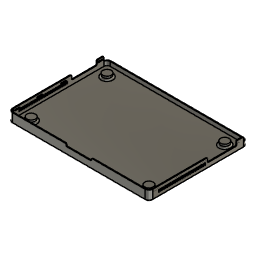
macbook case v2 (Autodesk Fusion 360 design; units mm, degrees)
Autodesk Fusion 360 part; units mm, degrees
note: some values were not read from the file. Chosen so that the rebuilt part matches the saved one: which bodies a step acts on.
sketch "Sketch1" plane through (0, 0, 0) normal (0, 0, 1) x (1, 0, 0)
  line L0 (93.5786, -68.8674) -> (-266.4214, -68.8674)
  line L1 (-266.4214, -68.8674) -> (-266.4214, 183.6326)
  line L2 (-266.4214, 183.6326) -> (93.5786, 183.6326)
  line L3 (93.5786, 183.6326) -> (93.5786, -68.8674)
  dimension "d1" = 360
  dimension "d2" = 252.5
  constraint horizontal L0
  constraint vertical L1
  constraint horizontal L2
  constraint vertical L3
  measures "d1" distance of L0.start L0.end
  measures "d2" distance of L0.start L2.end
extrude "Extrude1" add sketch "Sketch1" along normal blind 12.4 makes body 1
fillet "Fillet1" radius 10 4 edges at (-266.4214, 183.6326, 6.2) (-266.4214, -68.8674, 6.2) (93.5786, -68.8674, 6.2) (93.5786, 183.6326, 6.2) on bodies 1
shell "Shell1" thickness 2 removed faces 1 at (-143.0881, 99.466, 12.4) on bodies 1
chamfer "Chamfer1" distance 2 angle 45 8 edges at (93.5786, 57.3826, 0) (90.6497, -65.9384, 0) (-86.4214, -68.8674, 0) (-263.4925, -65.9384, 0) (-266.4214, 57.3826, 0) (-263.4925, 180.7037, 0) (-86.4214, 183.6326, 0) (90.6497, 180.7037, 0) on bodies 1
extrude "Extrude2" add 1 faces at (-29.7547, -68.2007, 12.4) along direction (0, 0, 1) blind 13 on bodies 1 bodies 1
sketch "Sketch2" plane through (0, 183.6326, 0) normal (0, 1, 0) x (-1, 0, 0)
  line L0 (-83.5786, 2) -> (256.4214, 2)
  line L1 (256.4214, 2) -> (256.4214, 25.4)
  line L2 (256.4214, 25.4) -> (-83.5786, 25.4)
  line L3 (-83.5786, 25.4) -> (-83.5786, 2)
  line L4 (-113.9565, 25.4) -> (284.3902, 25.4)
  line L5 (284.3902, 25.4) -> (284.3902, 13)
  line L6 (284.3902, 13) -> (-113.9565, 13)
  line L7 (-113.9565, 13) -> (-113.9565, 25.4)
  dimension "d11" = 12.4
  constraint horizontal L4
  constraint vertical L5
  constraint horizontal L6
  constraint vertical L7
  measures "d11" distance of L4.start L6.end
extrude "Extrude3" cut sketch "Sketch2" against normal blind 10 contours L3 L4 L6 L7 | L1 L2 L3 L4 L6 | L1 L4 L5 L6 bodies 1
sketch "Sketch3" plane through (-266.4214, 0, 0) normal (-1, 0, 0) x (0, -1, 0)
  line L0 (-173.6326, 2) -> (58.8674, 2)
  line L1 (58.8674, 2) -> (58.8674, 25.4)
  line L2 (58.8674, 25.4) -> (-173.6326, 25.4)
  line L3 (-173.6326, 25.4) -> (-173.6326, 13)
  line L4 (-173.6326, 13) -> (-173.6326, 2)
  line L5 (68.8674, 2) -> (68.8674, 25.4)
  line L6 (68.8674, 25.4) -> (-156.1326, 25.4) construction
  line L7 (-156.1326, 25.4) -> (-86.1326, 25.4)
  line L8 (-86.1326, 25.4) -> (-86.1326, 13)
  line L9 (-86.1326, 13) -> (-156.1326, 13)
  line L10 (-156.1326, 13) -> (-156.1326, 25.4)
  dimension "d14" = 225
  dimension "d15" = 70
  dimension "d16" = 12.4
  constraint coincident L5.end L6.start
  constraint perpendicular L1 L6
  constraint horizontal L7
  constraint vertical L8
  constraint horizontal L9
  constraint vertical L10
  measures "d14" distance of L5.end L6.end
  measures "d15" distance of L6.end L7.end
  measures "d16" distance of L6.end L9.end
extrude "Extrude4" cut sketch "Sketch3" against normal blind 30 contours L2 L7 L8 L9 L10 bodies 1
sketch "Sketch4" plane through (93.5786, 0, 0) normal (1, 0, 0) x (0, 1, 0)
  line L0 (-58.8674, 2) -> (173.6326, 2)
  line L1 (173.6326, 2) -> (173.6326, 13)
  line L2 (173.6326, 13) -> (173.6326, 25.4)
  line L3 (173.6326, 25.4) -> (-58.8674, 25.4)
  line L4 (-58.8674, 25.4) -> (-58.8674, 2)
  line L5 (-68.8674, 25.4) -> (-68.8674, 2)
  line L6 (-68.8674, 25.4) -> (156.1326, 25.4) construction
  line L7 (156.1326, 25.4) -> (81.1326, 25.4)
  line L8 (81.1326, 25.4) -> (81.1326, 13)
  line L9 (81.1326, 13) -> (156.1326, 13)
  line L10 (156.1326, 13) -> (156.1326, 25.4)
  dimension "d19" = 225
  dimension "d20" = 75
  dimension "d21" = 12.4
  constraint coincident L5.start L6.start
  constraint perpendicular L5 L6
  constraint horizontal L7
  constraint vertical L8
  constraint horizontal L9
  constraint vertical L10
  measures "d19" distance of L5.start L6.end
  measures "d20" distance of L6.end L7.end
  measures "d21" distance of L6.end L9.end
extrude "Extrude5" cut sketch "Sketch4" against normal blind 30 contours L3 L7 L8 L9 L10 bodies 1
sketch "Sketch5" plane through (93.5786, 0, 0) normal (1, 0, 0) x (0, 1, 0)
  line L0 (156.1326, 25.4) -> (156.1326, 13)
  line L1 (156.1326, 13) -> (81.1326, 13)
  line L2 (81.1326, 13) -> (81.1326, 25.4)
  line L3 (81.1326, 25.4) -> (-58.8674, 25.4)
  line L4 (-58.8674, 25.4) -> (-58.8674, 2)
  line L5 (-58.8674, 2) -> (173.6326, 2)
  line L6 (173.6326, 2) -> (173.6326, 13)
  line L7 (173.6326, 13) -> (173.6326, 25.4)
  line L8 (173.6326, 25.4) -> (156.1326, 25.4)
  line L9 (-68.8674, 25.4) -> (-68.8674, 2)
  line L10 (-68.8674, 25.4) -> (81.1326, 25.4) construction
  line L11 (6.1326, 25.4) -> (6.1326, 15.9) construction
  line L12 (-43.8674, 15.9) -> (81.1326, 15.9)
  line L13 (81.1326, 15.9) -> (81.1326, 9.9)
  line L14 (81.1326, 9.9) -> (-43.8674, 9.9)
  line L15 (-43.8674, 9.9) -> (-43.8674, 15.9)
  line L16 (-68.8674, 15.9) -> (-43.8674, 15.9) construction
  line L17 (-43.8674, 15.9) -> (-41.8674, 15.9)
  line L18 (-41.8674, 15.9) -> (-41.8674, 9.9)
  line L19 (-41.8674, 9.9) -> (-43.8674, 9.9)
  line L20 (-43.8674, 9.9) -> (-43.8674, 15.9)
  dimension "d24" = 150
  dimension "d25" = 9.5
  dimension "d26" = 125
  dimension "d27" = 6
  dimension "d28" = 25
  dimension "d29" = 2
  constraint coincident L9.start L10.start
  constraint perpendicular L4 L10
  constraint midpoint L10 L11.start
  constraint perpendicular L5 L11
  constraint horizontal L12
  constraint vertical L13
  constraint horizontal L14
  constraint vertical L15
  constraint coincident L9 L16.start
  constraint perpendicular L4 L16
  constraint coincident L12.start L15.end
  constraint horizontal L17
  constraint vertical L18
  constraint horizontal L19
  constraint vertical L20
  measures "d24" distance of L9.start L2.end
  measures "d25" distance of L11.start L11.end
  measures "d26" distance of L12.start L12.end
  measures "d27" distance of L12.start L14.end
  measures "d28" distance of L16.start L12.start
  measures "d29" distance of L12.start L17.end
extrude "Extrude6" cut sketch "Sketch5" against normal blind 460 contours L12 L14 L15 L17 L18 L19 L20 bodies 1
pattern_linear "R-Pattern1" count 30 spacing 4.2069 along (0, 1, 0) of "Extrude6"
extrude "Extrude7" add 1 faces at (-265.7547, 86.1326, 21.2667) along direction (0, 1, 0) blind 5 on bodies 1 bodies 1
sketch "Sketch6" plane through (93.5786, 0, 0) normal (1, 0, 0) x (0, 1, 0)
  line L0 (80.1326, 15.9) -> (80.1326, 9.9)
  line L1 (80.1326, 9.9) -> (78.1326, 9.9)
  line L2 (78.1326, 9.9) -> (78.1326, 15.9)
  line L3 (78.1326, 15.9) -> (80.1326, 15.9)
  line L4 (75.9257, 15.9) -> (75.9257, 9.9)
  line L5 (75.9257, 9.9) -> (73.9257, 9.9)
  line L6 (73.9257, 9.9) -> (73.9257, 15.9)
  line L7 (73.9257, 15.9) -> (75.9257, 15.9)
  line L8 (71.7188, 15.9) -> (71.7188, 9.9)
  line L9 (71.7188, 9.9) -> (69.7188, 9.9)
  line L10 (69.7188, 9.9) -> (69.7188, 15.9)
  line L11 (69.7188, 15.9) -> (71.7188, 15.9)
  line L12 (67.5119, 15.9) -> (67.5119, 9.9)
  line L13 (67.5119, 9.9) -> (65.5119, 9.9)
  line L14 (65.5119, 9.9) -> (65.5119, 15.9)
  line L15 (65.5119, 15.9) -> (67.5119, 15.9)
  line L16 (63.305, 15.9) -> (63.305, 9.9)
  line L17 (63.305, 9.9) -> (61.305, 9.9)
  line L18 (61.305, 9.9) -> (61.305, 15.9)
  line L19 (61.305, 15.9) -> (63.305, 15.9)
  line L20 (59.0981, 15.9) -> (59.0981, 9.9)
  line L21 (59.0981, 9.9) -> (57.0981, 9.9)
  line L22 (57.0981, 9.9) -> (57.0981, 15.9)
  line L23 (57.0981, 15.9) -> (59.0981, 15.9)
  line L24 (54.8912, 15.9) -> (54.8912, 9.9)
  line L25 (54.8912, 9.9) -> (52.8912, 9.9)
  line L26 (52.8912, 9.9) -> (52.8912, 15.9)
  line L27 (52.8912, 15.9) -> (54.8912, 15.9)
  line L28 (50.6844, 15.9) -> (50.6844, 9.9)
  line L29 (50.6844, 9.9) -> (48.6844, 9.9)
  line L30 (48.6844, 9.9) -> (48.6844, 15.9)
  line L31 (48.6844, 15.9) -> (50.6844, 15.9)
  line L32 (46.4775, 15.9) -> (46.4775, 9.9)
  line L33 (46.4775, 9.9) -> (44.4775, 9.9)
  line L34 (44.4775, 9.9) -> (44.4775, 15.9)
  line L35 (44.4775, 15.9) -> (46.4775, 15.9)
  line L36 (42.2706, 15.9) -> (42.2706, 9.9)
  line L37 (42.2706, 9.9) -> (40.2706, 9.9)
  line L38 (40.2706, 9.9) -> (40.2706, 15.9)
  line L39 (40.2706, 15.9) -> (42.2706, 15.9)
  line L40 (38.0637, 15.9) -> (38.0637, 9.9)
  line L41 (38.0637, 9.9) -> (36.0637, 9.9)
  line L42 (36.0637, 9.9) -> (36.0637, 15.9)
  line L43 (36.0637, 15.9) -> (38.0637, 15.9)
  line L44 (33.8568, 15.9) -> (33.8568, 9.9)
  line L45 (33.8568, 9.9) -> (31.8568, 9.9)
  line L46 (31.8568, 9.9) -> (31.8568, 15.9)
  line L47 (31.8568, 15.9) -> (33.8568, 15.9)
  line L48 (29.6499, 15.9) -> (29.6499, 9.9)
  line L49 (29.6499, 9.9) -> (27.6499, 9.9)
  line L50 (27.6499, 9.9) -> (27.6499, 15.9)
  line L51 (27.6499, 15.9) -> (29.6499, 15.9)
  line L52 (25.443, 15.9) -> (25.443, 9.9)
  line L53 (25.443, 9.9) -> (23.443, 9.9)
  line L54 (23.443, 9.9) -> (23.443, 15.9)
  line L55 (23.443, 15.9) -> (25.443, 15.9)
  line L56 (21.2361, 15.9) -> (21.2361, 9.9)
  line L57 (21.2361, 9.9) -> (19.2361, 9.9)
  line L58 (19.2361, 9.9) -> (19.2361, 15.9)
  line L59 (19.2361, 15.9) -> (21.2361, 15.9)
  line L60 (17.0292, 15.9) -> (17.0292, 9.9)
  line L61 (17.0292, 9.9) -> (15.0292, 9.9)
  line L62 (15.0292, 9.9) -> (15.0292, 15.9)
  line L63 (15.0292, 15.9) -> (17.0292, 15.9)
  line L64 (12.8223, 15.9) -> (12.8223, 9.9)
  line L65 (12.8223, 9.9) -> (10.8223, 9.9)
  line L66 (10.8223, 9.9) -> (10.8223, 15.9)
  line L67 (10.8223, 15.9) -> (12.8223, 15.9)
  line L68 (8.6154, 15.9) -> (8.6154, 9.9)
  line L69 (8.6154, 9.9) -> (6.6154, 9.9)
  line L70 (6.6154, 9.9) -> (6.6154, 15.9)
  line L71 (6.6154, 15.9) -> (8.6154, 15.9)
  line L72 (4.4085, 15.9) -> (4.4085, 9.9)
  line L73 (4.4085, 9.9) -> (2.4085, 9.9)
  line L74 (2.4085, 9.9) -> (2.4085, 15.9)
  line L75 (2.4085, 15.9) -> (4.4085, 15.9)
  line L76 (0.2016, 15.9) -> (0.2016, 9.9)
  line L77 (0.2016, 9.9) -> (-1.7984, 9.9)
  line L78 (-1.7984, 9.9) -> (-1.7984, 15.9)
  line L79 (-1.7984, 15.9) -> (0.2016, 15.9)
  line L80 (-4.0053, 15.9) -> (-4.0053, 9.9)
  line L81 (-4.0053, 9.9) -> (-6.0053, 9.9)
  line L82 (-6.0053, 9.9) -> (-6.0053, 15.9)
  line L83 (-6.0053, 15.9) -> (-4.0053, 15.9)
  line L84 (-8.2122, 15.9) -> (-8.2122, 9.9)
  line L85 (-8.2122, 9.9) -> (-10.2122, 9.9)
  line L86 (-10.2122, 9.9) -> (-10.2122, 15.9)
  line L87 (-10.2122, 15.9) -> (-8.2122, 15.9)
  line L88 (-12.4191, 15.9) -> (-12.4191, 9.9)
  line L89 (-12.4191, 9.9) -> (-14.4191, 9.9)
  line L90 (-14.4191, 9.9) -> (-14.4191, 15.9)
  line L91 (-14.4191, 15.9) -> (-12.4191, 15.9)
  line L92 (-16.626, 15.9) -> (-16.626, 9.9)
  line L93 (-16.626, 9.9) -> (-18.626, 9.9)
  line L94 (-18.626, 9.9) -> (-18.626, 15.9)
  line L95 (-18.626, 15.9) -> (-16.626, 15.9)
  line L96 (-20.8329, 15.9) -> (-20.8329, 9.9)
  line L97 (-20.8329, 9.9) -> (-22.8329, 9.9)
  line L98 (-22.8329, 9.9) -> (-22.8329, 15.9)
  line L99 (-22.8329, 15.9) -> (-20.8329, 15.9)
  line L100 (-25.0398, 15.9) -> (-25.0398, 9.9)
  line L101 (-25.0398, 9.9) -> (-27.0398, 9.9)
  line L102 (-27.0398, 9.9) -> (-27.0398, 15.9)
  line L103 (-27.0398, 15.9) -> (-25.0398, 15.9)
  line L104 (-29.2467, 15.9) -> (-29.2467, 9.9)
  line L105 (-29.2467, 9.9) -> (-31.2467, 9.9)
  line L106 (-31.2467, 9.9) -> (-31.2467, 15.9)
  line L107 (-31.2467, 15.9) -> (-29.2467, 15.9)
  line L108 (-33.4536, 15.9) -> (-33.4536, 9.9)
  line L109 (-33.4536, 9.9) -> (-35.4536, 9.9)
  line L110 (-35.4536, 9.9) -> (-35.4536, 15.9)
  line L111 (-35.4536, 15.9) -> (-33.4536, 15.9)
  line L112 (-37.6605, 15.9) -> (-37.6605, 9.9)
  line L113 (-37.6605, 9.9) -> (-39.6605, 9.9)
  line L114 (-39.6605, 9.9) -> (-39.6605, 15.9)
  line L115 (-39.6605, 15.9) -> (-37.6605, 15.9)
  line L116 (-41.8674, 15.9) -> (-41.8674, 9.9)
  line L117 (-41.8674, 9.9) -> (-43.8674, 9.9)
  line L118 (-43.8674, 9.9) -> (-43.8674, 15.9)
  line L119 (-43.8674, 15.9) -> (-41.8674, 15.9)
  line L120 (156.1326, 25.4) -> (156.1326, 13)
  line L121 (156.1326, 13) -> (81.1326, 13)
  line L122 (81.1326, 13) -> (81.1326, 25.4)
  line L123 (81.1326, 25.4) -> (-58.8674, 25.4)
  line L124 (-58.8674, 25.4) -> (-58.8674, 2)
  line L125 (-58.8674, 2) -> (173.6326, 2)
  line L126 (173.6326, 2) -> (173.6326, 13)
  line L127 (173.6326, 13) -> (173.6326, 25.4)
  line L128 (173.6326, 25.4) -> (156.1326, 25.4)
extrude "Extrude8" add sketch "Sketch6" against normal blind 2 contours L0 L1 L2 L3 bodies 1
sketch "Sketch7" plane through (0, -68.8674, 0) normal (0, -1, 0) x (1, 0, 0)
  line L0 (-256.4214, 2) -> (83.5786, 2)
  line L1 (83.5786, 2) -> (83.5786, 25.4)
  line L2 (83.5786, 25.4) -> (-256.4214, 25.4)
  line L3 (-256.4214, 25.4) -> (-256.4214, 2)
  line L4 (-118.9214, 25.4) -> (-53.9214, 25.4)
  line L5 (-53.9214, 25.4) -> (-53.9214, 18.4)
  line L6 (-53.9214, 18.4) -> (-118.9214, 18.4)
  line L7 (-118.9214, 18.4) -> (-118.9214, 25.4)
  dimension "d40" = 65
  dimension "d41" = 7
  constraint horizontal L4
  constraint vertical L5
  constraint horizontal L6
  constraint vertical L7
  constraint midpoint L2 L4
  measures "d40" distance of L4.start L4.end
  measures "d41" distance of L4.start L6.end
extrude "Extrude9" cut sketch "Sketch7" against normal blind 30 contours L2 L4 L5 L6 L7 bodies 1
sketch "Sketch8" plane through (0, 0, 2) normal (0, 0, 1) x (-1, 0, 0)
  arc A0 (-91.5786, -173.6326) -> (-83.5786, -181.6326) centre (-83.5786, -173.6326) ccw
  line L0 (-83.5786, -181.6326) -> (256.4214, -181.6326)
  arc A1 (256.4214, -181.6326) -> (264.4214, -173.6326) centre (256.4214, -173.6326) ccw
  line L1 (264.4214, -173.6326) -> (264.4214, 58.8674)
  arc A2 (264.4214, 58.8674) -> (256.4214, 66.8674) centre (256.4214, 58.8674) ccw
  line L2 (256.4214, 66.8674) -> (-83.5786, 66.8674)
  arc A3 (-83.5786, 66.8674) -> (-91.5786, 58.8674) centre (-83.5786, 58.8674) ccw
  line L3 (-91.5786, 58.8674) -> (-91.5786, -173.6326)
  line L4 (264.4214, -181.6326) -> (237.4214, -181.6326) construction
  line L5 (237.4214, -181.6326) -> (237.4214, -154.6326) construction
  line L6 (237.4214, -154.6326) -> (264.4214, -154.6326) construction
  line L7 (264.4214, -154.6326) -> (264.4214, -181.6326) construction
  line L8 (264.4214, 66.8674) -> (237.4214, 66.8674) construction
  line L9 (237.4214, 66.8674) -> (237.4214, 39.8674) construction
  line L10 (237.4214, 39.8674) -> (264.4214, 39.8674) construction
  line L11 (264.4214, 39.8674) -> (264.4214, 66.8674) construction
  line L12 (-91.5786, 66.8674) -> (-64.5786, 66.8674) construction
  line L13 (-64.5786, 66.8674) -> (-64.5786, 39.8674) construction
  line L14 (-64.5786, 39.8674) -> (-91.5786, 39.8674) construction
  line L15 (-91.5786, 39.8674) -> (-91.5786, 66.8674) construction
  line L16 (-91.5786, -181.6326) -> (-64.5786, -181.6326) construction
  line L17 (-64.5786, -181.6326) -> (-64.5786, -154.6326) construction
  line L18 (-64.5786, -154.6326) -> (-91.5786, -154.6326) construction
  line L19 (-91.5786, -154.6326) -> (-91.5786, -181.6326) construction
  circle A4 centre (-64.5786, -154.6326) radius 11
  circle A5 centre (237.4214, -154.6326) radius 11
  circle A6 centre (237.4214, 39.8674) radius 11
  circle A7 centre (-64.5786, 39.8674) radius 11
  dimension "d44" = 27
  dimension "d45" = 27
  dimension "d46" = 27
  dimension "d47" = 27
  dimension "d48" = 27
  dimension "d49" = 27
  dimension "d50" = 27
  dimension "d51" = 27
  dimension "d52" = 22
  dimension "d53" = 22
  dimension "d54" = 22
  dimension "d55" = 22
  constraint horizontal L4
  constraint vertical L5
  constraint horizontal L6
  constraint vertical L7
  constraint horizontal L8
  constraint vertical L9
  constraint horizontal L10
  constraint vertical L11
  constraint horizontal L12
  constraint vertical L13
  constraint horizontal L14
  constraint vertical L15
  constraint horizontal L16
  constraint vertical L17
  constraint horizontal L18
  constraint vertical L19
  constraint coincident L17.end L18.start
  constraint coincident L5.end L6.start
  constraint coincident L9.end L10.start
  constraint coincident L13.end L14.start
  measures "d44" distance of L4.start L4.end
  measures "d45" distance of L4.start L6.end
  measures "d46" distance of L8.start L8.end
  measures "d47" distance of L8.start L10.end
  measures "d48" distance of L12.start L12.end
  measures "d49" distance of L12.start L14.end
  measures "d50" distance of L16.start L16.end
  measures "d51" distance of L16.start L18.end
  measures "d52" diameter of A4
  measures "d53" diameter of A5
  measures "d54" diameter of A6
  measures "d55" diameter of A7
extrude "Extrude10" add sketch "Sketch8" along normal blind 8.7 contours A4 | A5 | A6 | A7 bodies 1
fillet "Fillet2" radius 4 4 edges at (74.8342, 150.6549, 2) (-227.1658, 150.6549, 2) (74.8342, -43.8451, 2) (-227.1658, -43.8451, 2) on bodies 1
extrude "Extrude11" cut 4 faces at (92.2453, -12.2007, 25.4) (-265.7547, 41.1326, 25.4) (-265.7547, 167.7993, 25.4) (92.9119, 167.7993, 25.4) along direction (0, 0, -1) blind 1 on bodies 1 bodies 1
fillet "Fillet3" radius 2 2 edges at (92.5786, 156.1326, 13) (92.5786, 81.1326, 13) on bodies 1
fillet "Fillet4" radius 2 2 edges at (-265.4214, 91.1326, 13) (-265.4214, 156.1326, 13) on bodies 1
fillet "Fillet5" radius 2 2 edges at (-53.9214, -67.8674, 18.4) (-118.9214, -67.8674, 18.4) on bodies 1
fillet "Fillet6" radius 2 2 edges at (-53.9214, -67.8674, 24.4) (-118.9214, -67.8674, 24.4) on bodies 1
fillet "Fillet7" radius 2 3 edges at (92.5786, 81.1326, 24.4) (92.5786, 156.1326, 24.4) (92.5786, 173.6326, 24.4) on bodies 1
fillet "Fillet8" radius 2 3 edges at (-265.4214, 91.1326, 24.4) (-265.4214, 156.1326, 24.4) (-265.4214, 173.6326, 24.4) on bodies 1
fillet "Fillet9" radius 2 2 edges at (-265.4214, 173.6326, 13) (92.5786, 173.6326, 13) on bodies 1
sketch "Sketch9" plane through (91.5786, 0, 0) normal (-1, 0, 0) x (0, -1, 0)
  arc A0 (-171.6326, 24.4) -> (-173.6326, 22.4) centre (-171.6326, 22.4) ccw
  line L0 (-173.6326, 22.4) -> (-173.6326, 15)
  line L1 (-173.6326, 15) -> (-173.6326, 2)
  line L2 (-173.6326, 2) -> (58.8674, 2)
  line L3 (58.8674, 2) -> (58.8674, 24.4)
  line L4 (58.8674, 24.4) -> (-79.1326, 24.4)
  arc A1 (-79.1326, 24.4) -> (-81.1326, 22.4) centre (-79.1326, 22.4) ccw
  line L5 (-81.1326, 22.4) -> (-81.1326, 15)
  arc A2 (-83.1326, 13) -> (-81.1326, 15) centre (-83.1326, 15) ccw
  line L6 (-83.1326, 13) -> (-154.1326, 13)
  arc A3 (-156.1326, 15) -> (-154.1326, 13) centre (-154.1326, 15) ccw
  line L7 (-156.1326, 15) -> (-156.1326, 22.4)
  arc A4 (-156.1326, 22.4) -> (-158.1326, 24.4) centre (-158.1326, 22.4) ccw
  line L8 (-158.1326, 24.4) -> (-171.6326, 24.4)
  line L9 (-75.9257, 9.9) -> (-75.9257, 15.9)
  line L10 (-75.9257, 15.9) -> (-73.9257, 15.9)
  line L11 (-73.9257, 15.9) -> (-73.9257, 9.9)
  line L12 (-73.9257, 9.9) -> (-75.9257, 9.9)
  line L13 (-71.7188, 9.9) -> (-71.7188, 15.9)
  line L14 (-71.7188, 15.9) -> (-69.7188, 15.9)
  line L15 (-69.7188, 15.9) -> (-69.7188, 9.9)
  line L16 (-69.7188, 9.9) -> (-71.7188, 9.9)
  line L17 (-67.5119, 9.9) -> (-67.5119, 15.9)
  line L18 (-67.5119, 15.9) -> (-65.5119, 15.9)
  line L19 (-65.5119, 15.9) -> (-65.5119, 9.9)
  line L20 (-65.5119, 9.9) -> (-67.5119, 9.9)
  line L21 (-63.305, 9.9) -> (-63.305, 15.9)
  line L22 (-63.305, 15.9) -> (-61.305, 15.9)
  line L23 (-61.305, 15.9) -> (-61.305, 9.9)
  line L24 (-61.305, 9.9) -> (-63.305, 9.9)
  line L25 (-59.0981, 9.9) -> (-59.0981, 15.9)
  line L26 (-59.0981, 15.9) -> (-57.0981, 15.9)
  line L27 (-57.0981, 15.9) -> (-57.0981, 9.9)
  line L28 (-57.0981, 9.9) -> (-59.0981, 9.9)
  line L29 (-54.8912, 9.9) -> (-54.8912, 15.9)
  line L30 (-54.8912, 15.9) -> (-52.8912, 15.9)
  line L31 (-52.8912, 15.9) -> (-52.8912, 9.9)
  line L32 (-52.8912, 9.9) -> (-54.8912, 9.9)
  line L33 (-50.6844, 9.9) -> (-50.6844, 15.9)
  line L34 (-50.6844, 15.9) -> (-48.6844, 15.9)
  line L35 (-48.6844, 15.9) -> (-48.6844, 9.9)
  line L36 (-48.6844, 9.9) -> (-50.6844, 9.9)
  line L37 (-46.4775, 9.9) -> (-46.4775, 15.9)
  line L38 (-46.4775, 15.9) -> (-44.4775, 15.9)
  line L39 (-44.4775, 15.9) -> (-44.4775, 9.9)
  line L40 (-44.4775, 9.9) -> (-46.4775, 9.9)
  line L41 (-42.2706, 9.9) -> (-42.2706, 15.9)
  line L42 (-42.2706, 15.9) -> (-40.2706, 15.9)
  line L43 (-40.2706, 15.9) -> (-40.2706, 9.9)
  line L44 (-40.2706, 9.9) -> (-42.2706, 9.9)
  line L45 (-38.0637, 9.9) -> (-38.0637, 15.9)
  line L46 (-38.0637, 15.9) -> (-36.0637, 15.9)
  line L47 (-36.0637, 15.9) -> (-36.0637, 9.9)
  line L48 (-36.0637, 9.9) -> (-38.0637, 9.9)
  line L49 (-33.8568, 9.9) -> (-33.8568, 15.9)
  line L50 (-33.8568, 15.9) -> (-31.8568, 15.9)
  line L51 (-31.8568, 15.9) -> (-31.8568, 9.9)
  line L52 (-31.8568, 9.9) -> (-33.8568, 9.9)
  line L53 (-29.6499, 9.9) -> (-29.6499, 15.9)
  line L54 (-29.6499, 15.9) -> (-27.6499, 15.9)
  line L55 (-27.6499, 15.9) -> (-27.6499, 9.9)
  line L56 (-27.6499, 9.9) -> (-29.6499, 9.9)
  line L57 (-25.443, 9.9) -> (-25.443, 15.9)
  line L58 (-25.443, 15.9) -> (-23.443, 15.9)
  line L59 (-23.443, 15.9) -> (-23.443, 9.9)
  line L60 (-23.443, 9.9) -> (-25.443, 9.9)
  line L61 (-21.2361, 9.9) -> (-21.2361, 15.9)
  line L62 (-21.2361, 15.9) -> (-19.2361, 15.9)
  line L63 (-19.2361, 15.9) -> (-19.2361, 9.9)
  line L64 (-19.2361, 9.9) -> (-21.2361, 9.9)
  line L65 (-17.0292, 9.9) -> (-17.0292, 15.9)
  line L66 (-17.0292, 15.9) -> (-15.0292, 15.9)
  line L67 (-15.0292, 15.9) -> (-15.0292, 9.9)
  line L68 (-15.0292, 9.9) -> (-17.0292, 9.9)
  line L69 (-12.8223, 9.9) -> (-12.8223, 15.9)
  line L70 (-12.8223, 15.9) -> (-10.8223, 15.9)
  line L71 (-10.8223, 15.9) -> (-10.8223, 9.9)
  line L72 (-10.8223, 9.9) -> (-12.8223, 9.9)
  line L73 (-8.6154, 9.9) -> (-8.6154, 15.9)
  line L74 (-8.6154, 15.9) -> (-6.6154, 15.9)
  line L75 (-6.6154, 15.9) -> (-6.6154, 9.9)
  line L76 (-6.6154, 9.9) -> (-8.6154, 9.9)
  line L77 (-4.4085, 9.9) -> (-4.4085, 15.9)
  line L78 (-4.4085, 15.9) -> (-2.4085, 15.9)
  line L79 (-2.4085, 15.9) -> (-2.4085, 9.9)
  line L80 (-2.4085, 9.9) -> (-4.4085, 9.9)
  line L81 (-0.2016, 9.9) -> (-0.2016, 15.9)
  line L82 (-0.2016, 15.9) -> (1.7984, 15.9)
  line L83 (1.7984, 15.9) -> (1.7984, 9.9)
  line L84 (1.7984, 9.9) -> (-0.2016, 9.9)
  line L85 (4.0053, 9.9) -> (4.0053, 15.9)
  line L86 (4.0053, 15.9) -> (6.0053, 15.9)
  line L87 (6.0053, 15.9) -> (6.0053, 9.9)
  line L88 (6.0053, 9.9) -> (4.0053, 9.9)
  line L89 (8.2122, 9.9) -> (8.2122, 15.9)
  line L90 (8.2122, 15.9) -> (10.2122, 15.9)
  line L91 (10.2122, 15.9) -> (10.2122, 9.9)
  line L92 (10.2122, 9.9) -> (8.2122, 9.9)
  line L93 (12.4191, 9.9) -> (12.4191, 15.9)
  line L94 (12.4191, 15.9) -> (14.4191, 15.9)
  line L95 (14.4191, 15.9) -> (14.4191, 9.9)
  line L96 (14.4191, 9.9) -> (12.4191, 9.9)
  line L97 (16.626, 9.9) -> (16.626, 15.9)
  line L98 (16.626, 15.9) -> (18.626, 15.9)
  line L99 (18.626, 15.9) -> (18.626, 9.9)
  line L100 (18.626, 9.9) -> (16.626, 9.9)
  line L101 (20.8329, 9.9) -> (20.8329, 15.9)
  line L102 (20.8329, 15.9) -> (22.8329, 15.9)
  line L103 (22.8329, 15.9) -> (22.8329, 9.9)
  line L104 (22.8329, 9.9) -> (20.8329, 9.9)
  line L105 (25.0398, 9.9) -> (25.0398, 15.9)
  line L106 (25.0398, 15.9) -> (27.0398, 15.9)
  line L107 (27.0398, 15.9) -> (27.0398, 9.9)
  line L108 (27.0398, 9.9) -> (25.0398, 9.9)
  line L109 (29.2467, 9.9) -> (29.2467, 15.9)
  line L110 (29.2467, 15.9) -> (31.2467, 15.9)
  line L111 (31.2467, 15.9) -> (31.2467, 9.9)
  line L112 (31.2467, 9.9) -> (29.2467, 9.9)
  line L113 (33.4536, 9.9) -> (33.4536, 15.9)
  line L114 (33.4536, 15.9) -> (35.4536, 15.9)
  line L115 (35.4536, 15.9) -> (35.4536, 9.9)
  line L116 (35.4536, 9.9) -> (33.4536, 9.9)
  line L117 (37.6605, 9.9) -> (37.6605, 15.9)
  line L118 (37.6605, 15.9) -> (39.6605, 15.9)
  line L119 (39.6605, 15.9) -> (39.6605, 9.9)
  line L120 (39.6605, 9.9) -> (37.6605, 9.9)
  line L121 (41.8674, 9.9) -> (41.8674, 15.9)
  line L122 (41.8674, 15.9) -> (43.8674, 15.9)
  line L123 (43.8674, 15.9) -> (43.8674, 9.9)
  line L124 (43.8674, 9.9) -> (41.8674, 9.9)
  line L125 (-10.1326, 24.4) -> (-10.1326, 18.7) construction
  line L126 (-76.696, 18.7) -> (58.8674, 18.7) construction
  line L127 (-164.8826, 24.4) -> (-164.8826, 18.7) construction
  line L128 (-76.696, 19.95) -> (-62.696, 19.95)
  line L129 (-62.696, 19.95) -> (-62.696, 17.45)
  line L130 (-62.696, 17.45) -> (-76.696, 17.45)
  line L131 (-76.696, 17.45) -> (-76.696, 19.95)
  line L132 (-76.696, 18.7) -> (-62.696, 18.7) construction
  line L133 (-15.9143, 17.45) -> (-15.9143, 19.95)
  line L134 (-15.9143, 18.7) -> (-1.9143, 18.7) construction
  line L135 (-15.9143, 19.95) -> (-1.9143, 19.95)
  line L136 (-1.9143, 17.45) -> (-15.9143, 17.45)
  line L137 (-1.9143, 19.95) -> (-1.9143, 17.45)
  line L138 (-171.8826, 17.45) -> (-171.8826, 19.95)
  line L139 (-171.8826, 18.7) -> (-157.8826, 18.7) construction
  line L140 (-171.8826, 19.95) -> (-157.8826, 19.95)
  line L141 (-157.8826, 17.45) -> (-171.8826, 17.45)
  line L142 (-157.8826, 19.95) -> (-157.8826, 17.45)
  line L143 (41.9217, 17.45) -> (41.9217, 19.95)
  line L144 (41.9217, 18.7) -> (55.9217, 18.7) construction
  line L145 (41.9217, 19.95) -> (55.9217, 19.95)
  line L146 (55.9217, 17.45) -> (41.9217, 17.45)
  line L147 (55.9217, 19.95) -> (55.9217, 17.45)
  dimension "d76" = 5.7
  dimension "d77" = 5.7
  dimension "d78" = 14
  dimension "d79" = 2.5
  dimension "d80" = 14
  dimension "d81" = 2.5
  dimension "d82" = 14
  dimension "d83" = 2.5
  dimension "d84" = 14
  dimension "d85" = 2.5
  constraint midpoint L4 L125.start
  constraint perpendicular L4 L125
  constraint coincident L3 L126.end
  constraint perpendicular L3 L126
  constraint midpoint L8 L127.start
  constraint perpendicular L8 L127
  constraint horizontal L128
  constraint vertical L129
  constraint horizontal L130
  constraint vertical L131
  constraint midpoint L131 L126.start
  constraint midpoint L129 L132.end
  constraint horizontal L135
  constraint vertical L137
  constraint horizontal L136
  constraint vertical L133
  constraint midpoint L134.start L133
  constraint midpoint L134.end L137
  constraint horizontal L140
  constraint vertical L142
  constraint horizontal L141
  constraint vertical L138
  constraint midpoint L139.start L138
  constraint midpoint L139.end L142
  constraint horizontal L145
  constraint vertical L147
  constraint horizontal L146
  constraint vertical L143
  constraint midpoint L144.start L143
  constraint midpoint L144.end L147
  constraint coincident L126.start L132.start
  constraint midpoint L126 L134
  constraint collinear L126 L144
  constraint midpoint L127.end L139
  measures "d76" distance of L125.start L125.end
  measures "d77" distance of L127.start L127.end
  measures "d78" distance of L128.start L128.end
  measures "d79" distance of L128.start L130.end
  measures "d80" distance of L133.end L135.end
  measures "d81" distance of L133.start L133.end
  measures "d82" distance of L138.end L140.end
  measures "d83" distance of L138.start L138.end
  measures "d84" distance of L143.end L145.end
  measures "d85" distance of L143.start L143.end
extrude "Extrude12" add sketch "Sketch9" along normal blind 1 draft -45 separate body contours L128 L129 L130 L131 | L133 L135 L136 L137 | L138 L140 L141 L142 | L143 L145 L146 L147 makes body 2 at (91.5786, 72.0293, 18.2833) makes body 3 at (91.5786, 11.2476, 18.2833) makes body 4 at (91.5786, 162.5493, 18.2833) makes body 5 at (91.5786, -46.5884, 18.2833)
ref_plane "WorkPlane1" through (-86.4214, 57.3826, 13.2) normal (1, 0, 0) x (0, 1, 0)
mirror "Mirror1" about plane through (-86.4214, 57.3826, 13.2) normal (1, 0, 0) of bodies 5 3 2 4 makes body 6 at (-264.4214, 72.0293, 18.2833) makes body 7 at (-264.4214, 11.2476, 18.2833) makes body 8 at (-264.4214, 162.5493, 18.2833) makes body 9 at (-264.4214, -46.5884, 18.2833)
combine "Combine1" operation add target body 1 tool bodies 2 3 4 5 6 7 8 9
